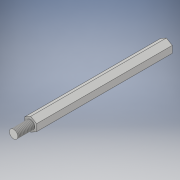
# Autodesk Inventor part: 六角支柱
Saved by Autodesk Inventor 2019 (Build 230136000, 136)
## iProperties
Created: 2020-09-20
Part Number: 六角支柱
Material: 一般
Document SubType Name: Modeling
Designer: Toshihito
Density: 1 g/cm^3
Appearance: 既定
Author: Toshihito
Autodesk Inventor part; units mm, degrees
ref_plane "YZ Plane" through (0, 0, 0) normal (1, 0, 0) x (0, 1, 0)
ref_plane "XZ Plane" through (0, 0, 0) normal (0, 1, 0) x (-1, 0, 0)
ref_plane "XY Plane" through (0, 0, 0) normal (0, 0, 1) x (1, 0, 0)
sketch "スケッチ1" plane through (0, 0, 0) normal (0, 0, 1) x (1, 0, 0)
  circle A0 centre (0, 0) radius 3.5
  line L0 (3.5, -2.0207) -> (0, -4.0415)
  line L1 (0, -4.0415) -> (-3.5, -2.0207)
  line L2 (-3.5, -2.0207) -> (-3.5, 2.0207)
  line L3 (-3.5, 2.0207) -> (0, 4.0415)
  line L4 (0, 4.0415) -> (3.5, 2.0207)
  line L5 (3.5, 2.0207) -> (3.5, -2.0207)
  point P0 (3.5, 0)
  dimension "d0" = 7
  constraints: 12 end point, 2 coincident, 1 horizontal alignment, 1 midpoint, 15 other
extrude "押し出し1" add sketch "スケッチ1" along normal blind 80
sketch "スケッチ2" plane through (0, 0, 80) normal (0, 0, 1) x (1, 0, 0)
  circle A0 centre (0, 0) radius 2.5
  dimension "d3" = 5
  constraints: 1 centre point, 1 coincident
  measures "d3" diameter of A0
sketch "スケッチ3" plane through (0, 0, 0) normal (0, 0, -1) x (-1, 0, 0)
  circle A0 centre (0, 0) radius 2.5
  dimension "d6" = 5
  constraints: 1 centre point, 1 coincident
  measures "d6" diameter of A0
extrude "押し出し3" cut sketch "スケッチ3" against normal blind 12
extrude "押し出し4" add sketch "スケッチ2" along normal blind 10
thread "ねじ1" size "M5x0.8" class "6g" standard "ANSI Metric M Profile" full length
